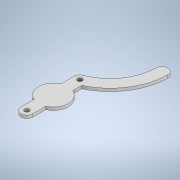
# Autodesk Inventor part: Pinzas
Saved by Autodesk Inventor 2021 (Build 250183000, 183)
## iProperties
Created: 2022-11-01
Part Number: Pinzas
Material: Generic
Document SubType Name: Modeling
Designer: USUARIO
Density: 1 g/cm^3
Appearance: Default
Author: USUARIO
Autodesk Inventor part; units mm, degrees
ref_plane "YZ Plane" through (0, 0, 0) normal (1, 0, 0) x (0, 1, 0)
ref_plane "XZ Plane" through (0, 0, 0) normal (0, 1, 0) x (-1, 0, 0)
ref_plane "XY Plane" through (0, 0, 0) normal (0, 0, 1) x (1, 0, 0)
sketch "Sketch1" plane through (0, 0, 0) normal (0, 1, 0) x (-1, 0, 0)
  line L0 (0, 45) -> (0, -45) construction
  line L1 (-10, 45) -> (-10, -45)
  line L2 (10, -45) -> (10, 45)
  arc A0 (10, 45) -> (-10, 45) centre (0, 45) ccw
  arc A1 (-10, -45) -> (10, -45) centre (0, -45) ccw
  circle A2 centre (0, 45) radius 4
  circle A3 centre (0, -45) radius 4
  arc A4 (0, -45) -> (-57.3576, -126.9152) centre (32.6209, -128.8801) ccw construction
  arc A5 (-3.6245, -35.68) -> (-67.3553, -126.6969) centre (32.6209, -128.8801) ccw
  arc A6 (3.6245, -54.32) -> (-47.36, -127.1335) centre (32.6209, -128.8801) ccw
  arc A7 (3.6245, -54.32) -> (-3.6245, -35.68) centre (0, -45) ccw
  arc A8 (-67.3553, -126.6969) -> (-47.36, -127.1335) centre (-57.3576, -126.9152) ccw
  line L3 (-57.3576, -126.9152) -> (0, -45)
  circle A9 centre (0, 0) radius 25
  point P0 (-5.7358, -53.1915)
  point P1 (10, -22.9129)
  point P2 (10, 22.9129)
  point P3 (-10, 22.9129)
  point P4 (-10, -22.9129)
  point P5 (-10, -38.4177)
  point P6 (-12.4556, -62.7885)
  point P7 (3.6245, -54.32)
  dimension "d0" = 20
  dimension "d2" = 90
  dimension "d3" = 8
  dimension "d4" = 8
  dimension "d5" = 20
  dimension "d7" = 100
  dimension "d8" = 145
  dimension "d9" = 100
  dimension "d10" = 50
  constraints: 14 point on circle, 10 centre point, 10 end point, 8 tangent, 5 coincident, 1 midpoint, 1 parallel, 1 vertical
  measures "d0" distance between parallel lines of L1 L2
  measures "d2" distance of L2.start L2.end
  measures "d3" diameter of A2
  measures "d4" diameter of A3
  measures "d5" radial gap between concentric circles of A5 A6
  measures "d7" distance of L3.start L0.end
  measures "d8" angle of L0 L3
  measures "d9" radius of A5
  measures "d10" diameter of A9
extrude "Extrusion1" add sketch "Sketch1" along normal blind 5 contours A0 L2 A9 L1 | A9 L2 L1 | L1 A9 | A9 L2 A7 A5 L1 | A9 L2 | A5 A7 A1 L1 | L1 A1 L3 A6 A8 A5 | A1 A6 L3
equation "\"d0\" = AnEsl"
equation "\"d5\" = AnEsl"
equation "\"d10\" = DV"
equation "\"DV\" = 50"
equation "\"AnEsl\" = 20"
body "Solid1"
